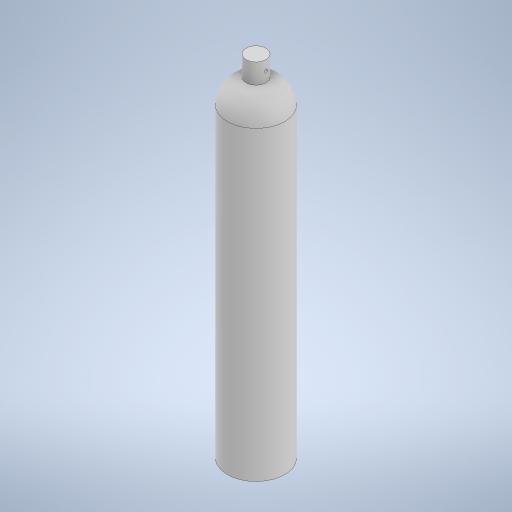
# Autodesk Inventor part: Cylinder
Saved by Autodesk Inventor 2024 (Build 280153020, 153B)
## iProperties
Created: 2023-08-30
Part Number: Cylinder
Material: Generic
Document SubType Name: Modeling
Designer: Victoria
Density: 1 g/cm^3
Appearance: Default
Author: Victoria
Autodesk Inventor part; units mm, degrees
ref_plane "YZ Plane" through (0, 0, 0) normal (1, 0, 0) x (0, 1, 0)
ref_plane "XZ Plane" through (0, 0, 0) normal (0, 1, 0) x (-1, 0, 0)
ref_plane "XY Plane" through (0, 0, 0) normal (0, 0, 1) x (1, 0, 0)
sketch "Sketch1" plane through (0, 0, 0) normal (0, 1, 0) x (-1, 0, 0)
  circle A0 centre (0, 0) radius 57.5
  dimension "d0" = 115
  constraints: 1 centre point, 1 coincident
  measures "d0" diameter of A0
extrude "Extrusion1" add sketch "Sketch1" along normal blind 660
sketch "Sketch2" plane through (0, 660, 0) normal (0, 1, 0) x (1, 0, 0)
  circle A0 centre (0, 0) radius 20
  dimension "d3" = 40
  constraints: 1 centre point, 1 coincident
  measures "d3" diameter of A0
extrude "Extrusion2" add sketch "Sketch2" along normal blind 40
fillet "Fillet1" radius 50 1 edges at (57.5, 660, 0)
sketch "Sketch3" plane through (0, 0, 0) normal (1, 0, 0) x (0, 1, 0)
  line L0 (700, -20) -> (700, 20) projected
  line L1 (700, -20) -> (680, -20)
  line L2 (660, -20) -> (700, -20) projected
  line L3 (680, -20) -> (680, 0)
  circle A0 centre (680, 0) radius 3.175
  point P0 (0, 0)
  dimension "d7" = 20
  dimension "d8" = 6.35
  constraints: 4 end point, 1 centre point, 1 coincident, 1 midpoint, 1 perpendicular
  measures "d7" distance of L0.start L1.end
  measures "d8" diameter of A0
extrude "Extrusion3" cut sketch "Sketch3" along normal blind 40
body "Solid1"
